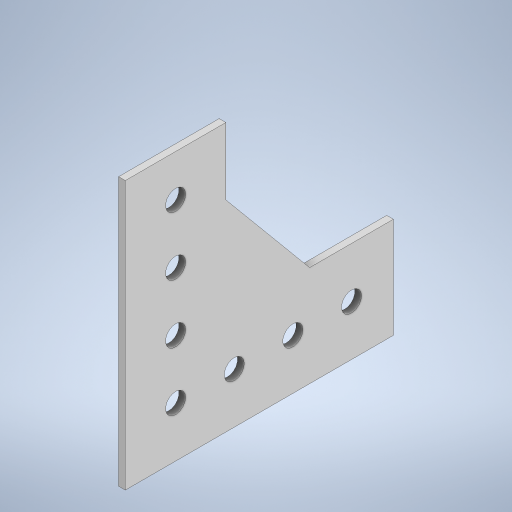
# Autodesk Inventor part: Connect2x3030_m6
Saved by Autodesk Inventor 2024 (Build 280153000, 153)
## iProperties
Created: 2025-12-08
Part Number: Connect2x3030_m6
Material: Generic
Document SubType Name: Modeling
Designer: schar
Density: 1 g/cm^3
Appearance: Default
Author: schar
Autodesk Inventor part; units mm, degrees
ref_plane "YZ Plane" through (0, 0, 0) normal (1, 0, 0) x (0, 1, 0)
ref_plane "XZ Plane" through (0, 0, 0) normal (0, 1, 0) x (-1, 0, 0)
ref_plane "XY Plane" through (0, 0, 0) normal (0, 0, 1) x (1, 0, 0)
sketch "Sketch4" plane through (0, 0, 0) normal (1, 0, 0) x (0, 1, 0)
  line L0 (0, 0) -> (80, 0)
  line L1 (80, 0) -> (80, -30)
  line L2 (80, -30) -> (0, -30)
  line L3 (0, -30) -> (0, 0)
  line L4 (0, -30) -> (30, -30)
  line L5 (30, -30) -> (30, -80)
  line L6 (30, -80) -> (0, -80)
  line L7 (0, -80) -> (0, -30)
  line L8 (80, -30) -> (60, -30)
  line L9 (60, -30) -> (30, -55)
  dimension "d10" = 80
  dimension "d11" = 30
  dimension "d12" = 30
  dimension "d13" = 50
  dimension "d14" = 20
  constraints: 20 end point, 4 parallel, 2 horizontal, 2 perpendicular, 1 midpoint, 1 point on line
  measures "d10" distance of L1.end L2.end
  measures "d11" distance of L0.end L1.end
  measures "d12" distance of L5.end L6.end
  measures "d13" distance of L4.end L5.end
  measures "d14" distance of L1.end L8.end
extrude "Extrusion2" add sketch "Sketch4" along normal blind 2
sketch "Sketch5" plane through (2, 0, 0) normal (1, 0, 0) x (0, 0, -1)
  line L0 (0, 80) -> (0, 0) projected
  line L1 (0, 0) -> (0, 15)
  line L2 (0, 15) -> (15, 15)
  circle A0 centre (15, 15) radius 3
  circle A1 centre (15, 32.5) radius 3
  circle A2 centre (15, 50) radius 3
  circle A3 centre (15, 67.5) radius 3
  circle A4 centre (32.5, 15) radius 3
  circle A5 centre (50, 15) radius 3
  circle A6 centre (67.5, 15) radius 3
  dimension "d17" = 15
  dimension "d18" = 15
  dimension "d22" = 6
  dimension "d25" = 17.5
  dimension "d35" = 17.5
  constraints: 7 centre point, 4 end point, 1 coincident, 1 horizontal, 1 perpendicular, 1 point on line, 1 vertical, 12 other
  measures "d17" distance of L0.end L1.end
  measures "d18" distance of L1.end L2.end
  measures "d22" diameter of A0
  measures "d25" distance of A0.centre A1.centre
  measures "d35" distance of A0.centre A4.centre
hole "Hole1" at (2, 67.5, -15) at (2, 50, -15) at (2, 32.5, -15) at (2, 15, -15) at (2, 15, -32.5) at (2, 15, -50) at (2, 15, -67.5) direction (-1, 0, 0) diameter 6 end through all
body "Solid2"
